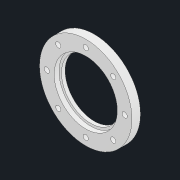
# Autodesk Inventor part: base8
Saved by Autodesk Inventor 2022 (Build 260153000, 153)
## iProperties
Created: 2021-09-17
Part Number: base8
Material: ABS プラスチック
Document SubType Name: Modeling
Designer: Yuta Kage
Density: 1.06 g/cm^3
Appearance: 滑らか - 白
Author: Yuta Kage
Autodesk Inventor part; units mm, degrees
ref_plane "YZ Plane" through (0, 0, 0) normal (1, 0, 0) x (0, 1, 0)
ref_plane "XZ Plane" through (0, 0, 0) normal (0, 1, 0) x (-1, 0, 0)
ref_plane "XY Plane" through (0, 0, 0) normal (0, 0, 1) x (1, 0, 0)
sketch "スケッチ1" plane through (0, 0, 0) normal (1, 0, 0) x (0, 1, 0)
  line L0 (24, 0) -> (38, 0)
  line L1 (38, 0) -> (38, 7)
  line L2 (38, 7) -> (26, 7)
  line L3 (26, 7) -> (26, 3)
  line L4 (26, 3) -> (24, 3)
  line L5 (24, 3) -> (24, 0)
  line L6 (0, -1.4) -> (0, 8.4) projected
  point P0 (0, 0)
  dimension "d0" = 24
  dimension "d1" = 38
  dimension "d2" = 26
  dimension "d3" = 4
  dimension "d5" = 3
  constraints: 13 end point, 5 perpendicular, 1 horizontal, 1 horizontal alignment
  measures "d0" distance from line of point (0, 0) L5
  measures "d1" distance from line of point (0, 0) L1
  measures "d2" distance from line of point (0, 0) L3
  measures "d3" distance of L2.end L3.end
  measures "d5" distance of L4.end L0.start
revolve "回転1" add sketch "スケッチ1" angle 360 about axis through (0, 0, -10) along (0, 0, 1)
sketch "スケッチ2" plane through (0, 0, 7) normal (0, 0, 1) x (1, 0, 0)
  circle A0 centre (0, 0) radius 32
  point P0 (0, 32)
  point P1 (-22.6274, 22.6274)
  point P2 (-32, 0)
  point P3 (-22.6274, -22.6274)
  point P4 (0, -32)
  point P5 (22.6274, -22.6274)
  point P6 (32, 0)
  point P7 (22.6274, 22.6274)
  dimension "d7" = 64
  dimension "d10" = 360
  constraints: 1 coincident, 1 vertical alignment, 11 other
hole "穴1" at (0, 32, 7) at (-22.6274, 22.6274, 7) at (-32, 0, 7) at (-22.6274, -22.6274, 7) at (0, -32, 7) at (22.6274, -22.6274, 7) at (32, 0, 7) at (22.6274, 22.6274, 7) direction (0, 0, -1) diameter 4.3 end through all clearance for "Socket Head Cap Screw" size "M4" standard "Ansi Metric M Profile"
